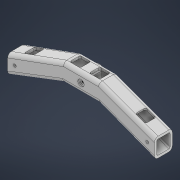
# Autodesk Inventor part: Fahrwerk_bogie
Saved by Autodesk Inventor 2021 (Build 250183000, 183)
## iProperties
Created: 2020-12-29
Part Number: Fahrwerk_bogie
Material: Generisch
Document SubType Name: Modeling
Designer: laure
Density: 1 g/cm^3
Appearance: Vorgabe
Author: laure
## iProperties of the stored document _3D-Druck.ipt
Created: 2021-01-28
Part Number: _3D-Druck
Material: Generisch
Document SubType Name: Modeling
Designer: Ctroi
Density: 1 g/cm^3
Appearance: Vorgabe
Author: Ctroi
Autodesk Inventor part; units mm, degrees
ref_plane "YZ Plane" through (0, 0, 0) normal (1, 0, 0) x (0, 1, 0)
ref_plane "XZ Plane" through (0, 0, 0) normal (0, 1, 0) x (-1, 0, 0)
ref_plane "XY Plane" through (0, 0, 0) normal (0, 0, 1) x (1, 0, 0)
sketch "Skizze1" plane through (0, 0, 0) normal (0, 0, 1) x (1, 0, 0)
  line L0 (-20, 10) -> (20, 10)
  line L1 (-20, 10) -> (-82.0197, -12.5733)
  line L2 (-20, 10) -> (46, 10) construction
  line L3 (-82.0197, -33.7893) -> (-20, -10)
  line L4 (20, 10) -> (82.0197, -12.5733)
  line L5 (20, 10) -> (86, 10) construction
  line L6 (82.0197, -33.7893) -> (20, -10)
  line L7 (-20, -10) -> (20, -10)
  line L8 (-82.0197, -12.5733) -> (-82.0197, -33.7893)
  line L9 (82.0197, -12.5733) -> (82.0197, -33.7893)
  line L10 (0, 18.7579) -> (0, -42.5472) projected
  line L11 (-115.6237, 0) -> (119.6039, 0) projected
  point P0 (0, 0)
  dimension "d0" = 40
  dimension "d3" = 66
  dimension "d7" = 66
  dimension "d8" = 20
  dimension "d87" = 10
  dimension "d89" = 20
  dimension "d92" = 10
  dimension "d95" = 40
  dimension "d106" = 21.216
  dimension "d107" = 21.216
  constraints: 20 end point, 4 horizontal, 2 equal length, 2 vertical, 1 symmetric about line, 2 other
  measures "d0" distance of L0.start L0.end
  measures "d3" distance of L0.start L1.end
  measures "d7" distance of L0.end L4.end
  measures "d8" angle of L4 L5
  measures "d87" distance between parallel lines of L0 L11
  measures "d89" angle of L1 L0
  measures "d92" distance between parallel lines of L11 L7
  measures "d95" distance of L3.end L6.end
  measures "d106" distance of L1.end L3.start
  measures "d107" distance of L4.end L6.start
extrude "Extrusion1" add sketch "Skizze1" along normal blind 20
fillet "Rundung3" radius 4 12 edges at (-51.0099, -1.2867, 20) (-51.0099, -1.2867, 0) (-51.0099, -21.8947, 20) (-51.0099, -21.8947, 0) (0, -10, 0) (0, -10, 20) (0, 10, 0) (51.0099, -1.2867, 0) (51.0099, -21.8947, 0) (51.0099, -21.8947, 20) (0, 10, 20) (51.0099, -1.2867, 20)
shell "Wandung3" thickness 2.6 removed faces 2 at (-82.0197, -25.2801, 13.3333) at (82.0197, -21.0551, 13.3333)
sketch "Skizze6" plane through (-82.0197, -12.5733, 16) normal (-0.3420201, 0.9396926, 0) x (0.9396926, 0.3420201, 0)
  line L0 (15, 12) -> (27, 12)
  line L1 (27, 12) -> (27, 0)
  line L2 (27, 0) -> (15, 0)
  line L3 (15, 0) -> (15, 12)
  line L4 (0, 12) -> (0, 0) projected
  line L5 (0, 12) -> (66, 12) projected
  line L6 (65.2947, 16) -> (-1.4559, 16) projected
  point P0 (81.3737, 16)
  dimension "d51" = 12
  dimension "d52" = 12
  dimension "d53" = 15
  dimension "d98" = 4
  constraints: 8 end point, 2 parallel, 1 horizontal, 1 perpendicular
  measures "d51" distance of L1.end L2.end
  measures "d52" distance of L0.end L1.end
  measures "d53" distance between parallel lines of L3 L4
  measures "d98" distance between parallel lines of L6 L0
extrude "Extrusion8" cut sketch "Skizze6" against normal blind 3
sketch "Skizze7" plane through (20, 10, 16) normal (0.3420201, 0.9396926, 0) x (0.9396926, -0.3420201, 0)
  line L0 (51, 0) -> (39, 0)
  line L1 (39, 0) -> (39, 12)
  line L2 (39, 12) -> (51, 12)
  line L3 (51, 12) -> (51, 0)
  line L4 (66, 12) -> (66, 0) projected
  line L5 (66, 0) -> (0, 0) projected
  line L6 (67.4559, 16) -> (0.7053, 16) projected
  point P0 (-15.3737, 16)
  dimension "d57" = 12
  dimension "d58" = 12
  dimension "d59" = 15
  dimension "d99" = 4
  constraints: 8 end point, 2 parallel, 1 horizontal, 1 perpendicular
  measures "d57" distance of L1.end L2.end
  measures "d58" distance of L0.end L1.end
  measures "d59" distance between parallel lines of L4 L3
  measures "d99" distance between parallel lines of L6 L2
extrude "Extrusion9" cut sketch "Skizze7" against normal blind 3
sketch "Skizze8" plane through (-20, 10, 4) normal (0, 1, 0) x (1, 0, 0)
  line L0 (3, 0) -> (15, 0)
  line L1 (15, 0) -> (15, -12)
  line L2 (15, -12) -> (3, -12)
  line L3 (3, -12) -> (3, 0)
  line L4 (0, 0) -> (40, 0) projected
  line L5 (0, 0) -> (0, -12) projected
  line L6 (25, 0) -> (37, 0)
  line L7 (37, 0) -> (37, -12)
  line L8 (37, -12) -> (25, -12)
  line L9 (25, -12) -> (25, 0)
  line L10 (40, 0) -> (40, -12) projected
  line L11 (39.2947, 4) -> (0.7053, 4) projected
  line L12 (39.2947, 4) -> (0.7053, 4) projected
  line L13 (0.7053, -16) -> (39.2947, -16) projected
  point P0 (20, 4)
  point P1 (13.9792, 4)
  point P2 (26.0208, 4)
  dimension "d63" = 12
  dimension "d64" = 12
  dimension "d66" = 3
  dimension "d67" = 12
  dimension "d68" = 12
  dimension "d70" = 3
  dimension "d117" = 4
  dimension "d118" = 4
  constraints: 16 end point, 4 parallel, 2 horizontal, 2 perpendicular
  measures "d63" distance of L1.end L2.end
  measures "d64" distance of L0.end L1.end
  measures "d66" distance between parallel lines of L5 L3
  measures "d67" distance of L7.end L8.end
  measures "d68" distance of L6.end L7.end
  measures "d70" distance between parallel lines of L10 L7
  measures "d117" distance between parallel lines of L13 L8
  measures "d118" distance between parallel lines of L13 L2
extrude "Extrusion10" cut sketch "Skizze8" against normal blind 3
fillet "Rundung7" radius 2 16 edges at (-56.2034, -4.5604, 16) (-67.4797, -8.6646, 16) (-67.4797, -8.6646, 4) (-56.2034, -4.5604, 4) (17, 8.7, 4) (-5, 8.7, 4) (5, 8.7, 16) (-17, 8.7, 16) (-17, 8.7, 4) (17, 8.7, 16) (-5, 8.7, 16) (5, 8.7, 4) (56.2034, -4.5604, 4) (67.4797, -8.6646, 16) (67.4797, -8.6646, 4) (56.2034, -4.5604, 16)
sketch "Skizze12" plane through (0, 0, 0) normal (0, 0, -1) x (-1, 0, 0)
  circle A0 centre (-74.0197, -20.2558) radius 1.6
  line L0 (-82.0197, -29.5052) -> (-82.0197, -16.83) projected
  line L1 (-82.0197, -29.5052) -> (-82.0197, -16.83) projected
  line L2 (-82.0197, -23.1676) -> (-59.4671, -14.9591)
  line L3 (-82.0197, -23.1676) -> (-58.0197, -23.1676) construction
  circle A1 centre (74.0197, -20.2558) radius 1.6
  line L4 (82.0197, -16.83) -> (82.0197, -29.5052) projected
  line L5 (82.0197, -16.83) -> (82.0197, -29.5052) projected
  line L6 (82.0197, -23.1676) -> (62.8081, -16.1752)
  line L7 (82.0197, -23.1676) -> (102.4643, -23.1676) construction
  point P0 (0, 0)
  dimension "d108" = 3.2
  dimension "d109" = 8
  dimension "d110" = 24
  dimension "d111" = 20
  dimension "d112" = 3.2
  dimension "d113" = 8
  dimension "d114" = 160
  constraints: 8 end point, 2 centre point, 2 equal length, 2 horizontal, 2 midpoint, 2 point on line
  measures "d108" diameter of A0
  measures "d109" distance from line of L0 A0.centre
  measures "d110" distance of L2.start L2.end
  measures "d111" angle of L3 L2
  measures "d112" diameter of A1
  measures "d113" distance from line of A1.centre L4
  measures "d114" angle of L7 L6
extrude "Extrusion14" cut sketch "Skizze12" against normal up to surface (20 mm away)
sketch "Skizze14" plane through (20.7408, -6, 17.4) normal (0, 0, -1) x (-1, 0, 0)
  line L0 (14.7408, 12) -> (26.7408, 12)
  line L1 (26.7408, 12) -> (26.7408, 0)
  line L2 (26.7408, 0) -> (14.7408, 0)
  line L3 (14.7408, 0) -> (14.7408, 12)
  line L4 (20.7408, -36.5472) -> (20.7408, 24.7579) projected
  line L5 (-94.0868, 6) -> (135.5684, 6) projected
  point P0 (16.2408, 10.5)
  point P1 (25.2408, 1.5)
  dimension "d125" = 12
  dimension "d126" = 12
  constraints: 8 end point, 2 parallel, 1 horizontal, 1 perpendicular, 2 other
  measures "d125" distance between parallel lines of L1 L3
  measures "d126" distance between parallel lines of L2 L0
extrude "Extrusion17" add sketch "Skizze14" along normal up to surface (14.8 mm away)
sketch "Skizze13" plane through (0, 0, 0) normal (0, 0, -1) x (-1, 0, 0)
  line L0 (-4.5, 4.5) -> (4.5, 4.5)
  line L1 (4.5, 4.5) -> (4.5, -4.5)
  line L2 (4.5, -4.5) -> (-4.5, -4.5)
  line L3 (-4.5, -4.5) -> (-4.5, 4.5)
  line L4 (-4.5, 4.5) -> (4.5, -4.5) construction
  line L5 (4.5, 4.5) -> (-4.5, -4.5) construction
  point P0 (0, 0)
  dimension "d119" = 9
  dimension "d120" = 9
  constraints: 12 end point, 2 midpoint, 2 parallel, 1 horizontal, 1 perpendicular
  measures "d119" distance of L1.end L2.end
  measures "d120" distance of L0.end L1.end
extrude "Extrusion18" cut sketch "Skizze13" against normal up to surface (17.4 mm away)
sketch "Skizze15" plane through (0, 0, 20) normal (0, 0, 1) x (1, 0, 0)
  circle A0 centre (0, 0) radius 3.5
  dimension "d131" = 7
  constraints: 1 centre point, 1 coincident
  measures "d131" diameter of A0
extrude "Extrusion19" cut sketch "Skizze15" against normal blind 1
sketch "Skizze16" plane through (0, 0, 19) normal (0, 0, 1) x (1, 0, 0)
  circle A0 centre (0, 0) radius 3.5 projected
  circle A1 centre (0, 0) radius 1.6
  dimension "d134" = 3.2
  constraints: 1 centre point, 1 coincident
  measures "d134" diameter of A1
extrude "Extrusion20" cut sketch "Skizze16" against normal up to surface (1.6 mm away) contours A1
sketch "Skizze17" plane through (0, 0, 0) normal (0, 0, -1) x (-1, 0, 0)
  circle A0 centre (0, 0) radius 1.6 projected
  line L0 (-6, -6) -> (-6, 6) projected
  line L1 (-6, 6) -> (6.0208, 6)
  line L2 (19.2947, 6) -> (-19.2947, 6) projected
  line L3 (-20.7408, -6) -> (20.7408, -6) projected
  line L4 (6.0208, -6) -> (-6.0208, -6)
  arc A1 (-6.0208, -6) -> (6.0208, -6) centre (0, 0) ccw
  arc A2 (6.0208, 6) -> (-6.0208, 6) centre (0, 0) ccw
  dimension "d138" = 8.5
  dimension "d139" = 8.5
  constraints: 4 end point, 4 point on circle, 4 point on line, 2 centre point, 1 coincident
  measures "d138" radius of A2
  measures "d139" radius of A1
extrude "Extrusion21" add sketch "Skizze17" against normal blind 1 contours L2 A2 L1 | L3 A1
